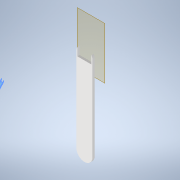
# Autodesk Inventor part: Brazo1
Saved by Autodesk Inventor 2022 (Build 260153000, 153)
## iProperties
Created: 2021-09-09
Part Number: Brazo1
Material: Generic
Document SubType Name: Modeling
Designer: Administrador
Density: 1 g/cm^3
Appearance: Default
Author: Administrador
Autodesk Inventor part; units mm, degrees
ref_plane "YZ Plane" through (0, 0, 0) normal (1, 0, 0) x (0, 1, 0)
ref_plane "XZ Plane" through (0, 0, 0) normal (0, 1, 0) x (-1, 0, 0)
ref_plane "XY Plane" through (0, 0, 0) normal (0, 0, 1) x (1, 0, 0)
ref_plane "Work Plane1" through (0, 0, 0) normal (0, 0, 1) x (1, 0, 0)
sketch "Sketch1" plane through (0, 0, 0) normal (0, 0, 1) x (1, 0, 0)
  line L0 (22.5, 14) -> (1.5, 14) projected
  line L1 (22.5, 56) -> (22.5, 14) projected
  line L2 (1.5, 56) -> (22.5, 56) projected
  line L3 (1.5, 14) -> (1.5, 56) projected
  line L4 (12, -3.3703) -> (12, 20.3) construction
  line L5 (12, 20.3) -> (1.5, 20.3) construction
  arc A0 (0, -104.7) -> (24, -104.7) centre (12, -104.7) ccw
  line L6 (0, -104.7) -> (0, 20.3)
  line L7 (24, -104.7) -> (24, 20.3)
  arc A1 (24, 20.3) -> (0, 20.3) centre (12, 20.3) ccw
  point P0 (0, 0)
  point P1 (1.5, 26.1095)
  point P2 (22.5, 26.1095)
  dimension "d2" = 10.5
  dimension "d4" = 6.3
  dimension "d6" = 24
  constraints: 8 end point, 4 point on circle, 3 tangent, 2 centre point, 1 perpendicular, 1 point on line, 1 vertical
  measures "d2" distance of L4.end L5.end
  measures "d4" distance from line of L4.end L0
  measures "d6" diameter of A0
extrude "Extrusion1" add sketch "Sketch1" along normal blind 3.3 contours L1 A1 L7 A0 L6 L3 L0 | L0 L3 A1 L1
body "Solid1"
